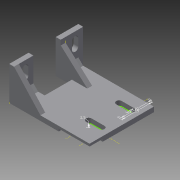
# Autodesk Inventor part: bart z endstop bracket v12
Saved by Autodesk Inventor 2014 SP1 (Build 180222100, 222)
## iProperties
Created: 2015-07-08
Part Number: bart z endstop bracket v12
Material: Generic
Document SubType Name: Modeling
Designer: Mon
Density: 1 g/cm^3
Appearance: Default
Author: Mon
Autodesk Inventor part; units mm, degrees
ref_plane "YZ Plane" through (0, 0, 0) normal (1, 0, 0) x (0, 1, 0)
ref_plane "XZ Plane" through (0, 0, 0) normal (0, 1, 0) x (-1, 0, 0)
ref_plane "XY Plane" through (0, 0, 0) normal (0, 0, 1) x (1, 0, 0)
sketch "Sketch1" plane through (0, 0, 0) normal (0, 0, 1) x (1, 0, 0)
  line L0 (0, 0) -> (50, 0)
  line L1 (50, 0) -> (50, -40)
  line L2 (50, -40) -> (0, -40)
  line L3 (0, -40) -> (0, 0)
  dimension "d0" = 50
  dimension "d1" = 40
  constraints: 8 end point, 2 parallel, 1 horizontal, 1 perpendicular
  measures "d0" distance of L1.end L2.end
  measures "d1" distance of L0.end L1.end
extrude "Extrusion1" add sketch "Sketch1" along normal blind 3
sketch "Sketch2" plane through (0, 0, 3) normal (0, 0, 1) x (1, 0, 0)
  line L0 (0, -40) -> (50, -40) projected
  line L1 (0, 0) -> (3, 0)
  line L2 (3, 0) -> (3, -40)
  line L3 (3, -40) -> (0, -40)
  line L4 (0, -40) -> (0, 0)
  dimension "d4" = 3
  constraints: 8 end point, 2 parallel, 1 horizontal, 1 perpendicular, 1 point on line
  measures "d4" distance of L2.end L3.end
extrude "Extrusion2" add sketch "Sketch2" along normal blind 18
sketch "Sketch3" plane through (0, 0, 0) normal (0, 1, 0) x (1, 0, 0)
  line L0 (0, 0) -> (3, 0)
  line L1 (3, 0) -> (3, -21)
  line L2 (3, -21) -> (0, -21)
  line L3 (0, -21) -> (0, 0)
  constraints: 8 end point, 2 parallel, 1 horizontal, 1 perpendicular
extrude "Extrusion3" add sketch "Sketch3" along normal blind 3
sketch "Sketch4" plane through (0, 0, 0) normal (0, 0, -1) x (-1, 0, 0)
  line L0 (0, -40) -> (0, 3) projected
  line L1 (-3, 0) -> (-3, 3) projected
  line L2 (-3, 0) -> (-3, -11)
  line L3 (0, -11) -> (-10, -11)
  line L4 (-10, -11) -> (-10, -27.9486)
  line L5 (-10, -27.9486) -> (0, -27.9486)
  point P0 (0, 0)
  dimension "d9" = 11
  dimension "d10" = 10
  constraints: 8 end point, 2 perpendicular, 2 point on line, 1 collinear, 1 parallel
  measures "d9" distance of L1.start L2.end
  measures "d10" distance of L3.start L3.end
extrude "Extrusion4" cut sketch "Sketch4" against normal blind 8
sketch "Sketch6" plane through (0, -40, 0) normal (-1, 0, 0) x (0, 0, 1)
  line L0 (0, 29) -> (8, 29) projected
  line L1 (12, 38) -> (16.5475, 38) construction
  line L2 (12, 36) -> (16.5475, 36)
  line L3 (16.5475, 40) -> (12, 40)
  arc A0 (12, 40) -> (12, 36) centre (12, 38) ccw
  arc A1 (16.5475, 36) -> (16.5475, 40) centre (16.5475, 38) ccw
  point P0 (0, 40)
  point P1 (14.2738, 38)
  constraints: 8 end point, 4 point on circle, 4 tangent, 2 centre point, 2 parallel, 1 midpoint
extrude "Extrusion6" cut sketch "Sketch6" against normal through all
sketch "Sketch7" plane through (0, -40, 0) normal (-1, 0, 0) x (0, 0, 1)
  line L0 (16.5475, 36) -> (12, 36) projected
  line L1 (12, 7) -> (16.5475, 7) construction
  line L2 (12, 5) -> (16.5475, 5)
  line L3 (16.5475, 9) -> (12, 9)
  arc A0 (12, 9) -> (12, 5) centre (12, 7) ccw
  arc A1 (16.5475, 5) -> (16.5475, 9) centre (16.5475, 7) ccw
  point P0 (0, 40)
  point P1 (14.2738, 7)
  dimension "d67" = 4
  constraints: 8 end point, 4 point on circle, 4 tangent, 2 centre point, 2 parallel, 1 midpoint
  measures "d67" diameter of A1
extrude "Extrusion7" cut sketch "Sketch7" against normal through all
sketch "Sketch8" plane through (0, 0, 0) normal (0, 0, -1) x (-1, 0, 0)
  line L0 (-45, -8.75) -> (-37, -8.75) construction
  line L1 (-45, -10.5) -> (-37, -10.5)
  line L2 (-37, -7) -> (-45, -7)
  arc A0 (-45, -7) -> (-45, -10.5) centre (-45, -8.75) ccw
  arc A1 (-37, -10.5) -> (-37, -7) centre (-37, -8.75) ccw
  line L3 (-10, -27.9486) -> (-10, -11) projected
  line L4 (-41, -8.75) -> (-41, -4.75) construction
  line L5 (-41, -4.75) -> (-35.5779, -4.75) construction
  point P0 (0, 0)
  dimension "d27" = 8
  dimension "d28" = 3.5
  dimension "d60" = 4
  constraints: 12 end point, 4 point on circle, 4 tangent, 2 centre point, 2 parallel, 1 midpoint, 1 perpendicular
  measures "d27" distance of L0.start L0.end
  measures "d28" diameter of A1
  measures "d60" distance of L4.start L4.end
extrude "Extrusion8" cut sketch "Sketch8" against normal through all
chamfer "Chamfer1" distance 3 angle 45 1 edges at (3, -33.9743, 3)
chamfer "Chamfer2" distance 3 angle 45 1 edges at (3, -5.5, 3)
sketch "Sketch11" plane through (0, 0, 0) normal (0, 0, -1) x (-1, 0, 0)
  line L0 (-10, -27.9486) -> (-10, -11) projected
  line L1 (-41.0188, 5.0018) -> (-41.0188, -13.9982) construction
  line L2 (-48.6932, -22.9665) -> (-25.0226, -22.9665) construction
  line L3 (-45, -41.7147) -> (-45, -21.8236) construction
  line L4 (-37, -41.7147) -> (-37, -21.8236) construction
  line L5 (-45, -22.9665) -> (-37, -22.9665) construction
  line L6 (-45, -29.2482) -> (-37, -29.2482)
  arc A0 (-45, -25.7482) -> (-45, -29.2482) centre (-45, -27.4982) ccw
  arc A1 (-37, -29.2482) -> (-37, -25.7482) centre (-37, -27.4982) ccw
  line L7 (0, -27.9486) -> (-10, -27.9486) projected
  line L8 (-41.0188, -8.7165) -> (-41.0188, -4.7165)
  line L9 (-41.0188, -4.7165) -> (-38.5918, -4.7165)
  line L10 (0, -40) -> (0, -27.9486) projected
  line L11 (-41.0188, 5.7518) -> (-41.0188, -13.2482) construction
  line L12 (-41.0188, -27.7165) -> (-56.6295, -27.7165) construction
  line L13 (-37, -25.7482) -> (-45, -25.7482)
  point P0 (0, 0)
  point P1 (-41, -22.9665)
  dimension "d43" = 19
  dimension "d44" = 3.5
  dimension "d59" = 4
  dimension "d61" = 19
  constraints: 22 end point, 5 perpendicular, 5 point on circle, 4 parallel, 3 point on line, 3 tangent, 2 centre point, 1 midpoint
  measures "d43" distance of L1.start L1.end
  measures "d44" diameter of A1
  measures "d59" distance of L8.start L8.end
  measures "d61" distance of L11.start L11.end
extrude "Extrusion11" cut sketch "Sketch11" against normal through all
sketch "Sketch12" plane through (0, 0, 0) normal (0, 0, -1) x (-1, 0, 0)
  line L0 (-10, -27.9486) -> (-10, -11) projected
  line L1 (-41, -25.8493) -> (-41, -31.8493) construction
  line L2 (-41, -31.8493) -> (-30.8265, -31.8493) construction
  line L3 (-30.8265, -31.8493) -> (-30.8265, -35.8493) construction
  line L4 (-30.8265, -35.8493) -> (-30.8265, -31.8493) construction
  line L5 (-30.8265, -31.8493) -> (-50, -31.8493)
  line L6 (-50, -31.8493) -> (-50, -40)
  line L7 (-50, -40) -> (-30.8265, -40)
  line L8 (-30.8265, -40) -> (-30.8265, -31.8493)
  point P0 (0, 0)
  dimension "d47" = 6
  dimension "d48" = 4
  dimension "d49" = 4
  constraints: 16 end point, 5 parallel, 2 perpendicular, 1 horizontal
  measures "d47" distance of L1.start L1.end
  measures "d48" distance of L2.end L3.end
  measures "d49" distance of L3.end L4.end
extrude "Extrusion12" cut sketch "Sketch12" against normal blind 1.5
sketch "Sketch13" plane through (0, 0, 0) normal (0, 0, -1) x (-1, 0, 0)
  line L0 (-45, -21.2165) -> (-37, -21.2165) projected
  arc A0 (-37, -10.5) -> (-37, -7) centre (-37, -8.75) ccw projected
  arc A1 (-45, -7) -> (-45, -10.5) centre (-45, -8.75) ccw projected
  line L1 (-45, -7) -> (-37, -7) projected
  line L2 (-46.75, -8.75) -> (-40.75, -8.75) construction
  line L3 (-40.75, -8.75) -> (-40.75, -24.7606) construction
  line L4 (-40.75, -24.7606) -> (-37.75, -24.7606) construction
  line L5 (-37.75, -11.2484) -> (-40.75, -11.2484) construction
  line L6 (-35.25, -8.75) -> (-29.25, -8.75) construction
  line L7 (-29.25, -8.75) -> (-29.25, -11.925) construction
  line L8 (-40.8665, -21.2165) -> (-40.75, -19.2199) construction
  line L9 (-29.25, -11.925) -> (-40.75, -11.925)
  line L10 (-40.75, -11.925) -> (-40.75, -24.7606)
  line L11 (-40.75, -24.7606) -> (-29.25, -24.7606)
  line L12 (-29.25, -24.7606) -> (-29.25, -11.925)
  point P0 (0, 0)
  point P1 (-40.75, -11.925)
  dimension "d52" = 6
  dimension "d53" = 3
  dimension "d54" = 6
  dimension "d55" = 3.175
  dimension "d56" = 2
  constraints: 22 end point, 5 parallel, 4 perpendicular, 4 point on line, 2 point on circle, 1 horizontal
  measures "d52" distance of L2.start L2.end
  measures "d53" distance of L3.end L4.end
  measures "d54" distance of L6.start L6.end
  measures "d55" distance of L6.end L7.end
  measures "d56" distance of L8.start L8.end
extrude "Extrusion13" cut sketch "Sketch13" against normal blind 1.5
ref_plane "Work Plane1" through (0, -8, 0) normal (0, 1, 0) x (1, 0, 0)
sketch "Sketch14" plane through (0, -8, 0) normal (0, 1, 0) x (1, 0, 0)
  line L0 (3.0794, -17.957) -> (19.7008, -2.8939)
  line L1 (19.7008, -2.8939) -> (3.0794, -2.8939)
  line L2 (3.0794, -2.8939) -> (3.0794, -17.957)
  point P0 (0, 0)
  constraints: 6 end point, 1 horizontal, 1 perpendicular
extrude "Extrusion14" add sketch "Sketch14" against normal blind 3
sketch "Sketch15" plane through (0, -40, 21) normal (0, -1, 0) x (1, 0, 0)
  line L0 (6, -18) -> (50, -18) projected
  line L1 (3, -15) -> (6, -18) projected
  line L2 (3, -15) -> (3, 0) projected
  line L3 (3, 0) -> (19.3977, -18)
  line L4 (3, -15.75) -> (3, 0)
  constraints: 4 end point, 1 collinear, 1 point on line
extrude "Extrusion15" add sketch "Sketch15" against normal blind 3
sketch "Sketch16" plane through (3, 0, 0) normal (1, 0, 0) x (0, 0, -1)
  line L0 (-21, -37) -> (-21, 3) projected
  line L1 (-21, -11) -> (-8, -11)
  line L2 (-8, -11) -> (-8, -27.9486)
  line L3 (-8, -27.9486) -> (-21, -27.9486)
  line L4 (-21, -27.9486) -> (-21, -11)
  constraints: 8 end point, 2 parallel, 1 horizontal, 1 perpendicular, 1 point on line
extrude "Extrusion16" cut sketch "Sketch16" against normal through all
body "Solid1"
